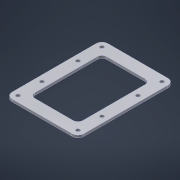
# Autodesk Inventor part: P018-Joint_carter_chapeau
Saved by Autodesk Inventor 2021.3 (Build 253353000, 353)
## iProperties
Created: 2022-05-28
Part Number: P018-Joint_carter_chapeau
Material: Polytetrafluoroethylene
Document SubType Name: Modeling
Designer: Rémi Heredero
Density: 2.02 g/cm^3
Appearance: PTFE
Mass: 9.3425 g
Surface Area: 57.3079 cm^2
Volume: 4.625 cm^3
Author: Rémi Heredero
Autodesk Inventor part; units mm, degrees
ref_plane "YZ Plane" through (0, 0, 0) normal (1, 0, 0) x (0, 1, 0)
ref_plane "XZ Plane" through (0, 0, 0) normal (0, 1, 0) x (-1, 0, 0)
ref_plane "XY Plane" through (0, 0, 0) normal (0, 0, 1) x (1, 0, 0)
sketch "Sketch2" plane through (0, 0, 0) normal (0, 0, 1) x (1, 0, 0)
  circle A0 centre (25, -25) radius 1.621 projected
  circle A1 centre (-25, 5) radius 1.621 projected
  circle A2 centre (-25, 25) radius 1.621 projected
  circle A3 centre (25, -45) radius 1.621 projected
  circle A4 centre (-25, -45) radius 1.621 projected
  circle A5 centre (25, 25) radius 1.621 projected
  circle A6 centre (-25, -25) radius 1.621 projected
  circle A7 centre (25, 5) radius 1.621 projected
  line L0 (30, -45) -> (30, 25) projected
  line L1 (25, 30) -> (-25, 30) projected
  line L2 (-30, 25) -> (-30, -45) projected
  line L3 (-25, -50) -> (25, -50) projected
  line L4 (16, -40) -> (-16, -40) projected
  line L5 (-20, -36) -> (-20, 16) projected
  line L6 (-16, 20) -> (16, 20) projected
  line L7 (20, 16) -> (20, -36) projected
  arc A8 (-30, -45) -> (-25, -50) centre (-25, -45) ccw projected
  arc A9 (25, -50) -> (30, -45) centre (25, -45) ccw projected
  arc A10 (30, 25) -> (25, 30) centre (25, 25) ccw projected
  arc A11 (-25, 30) -> (-30, 25) centre (-25, 25) ccw projected
  arc A12 (-20, -36) -> (-16, -40) centre (-16, -36) ccw projected
  arc A13 (-16, 20) -> (-20, 16) centre (-16, 16) ccw projected
  arc A14 (20, 16) -> (16, 20) centre (16, 16) ccw projected
  arc A15 (16, -40) -> (20, -36) centre (16, -36) ccw projected
extrude "Extrusion1" add sketch "Sketch2" against normal blind 2
body "Solid1"
